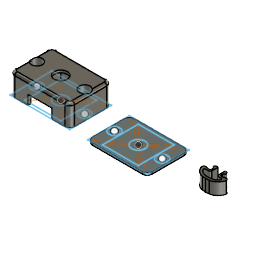
CNC Spindle speed control potentiometer box (Autodesk Fusion 360 design; units mm, degrees)
part number: 2025-11-11-00-48-20-010
Autodesk Fusion 360 part; units mm, degrees
other "Base Mesh Feature1"
sketch "Sketch1" plane through (0, 0, 0) normal (0, 0, 1) x (1, 0, 0)
other "Modify1"
sketch "Sketch2" plane through (0, 0, 0) normal (0, 0, 1) x (1, 0, 0)
  line L0 (5.2002, 7.2077) -> (5.2002, 2)
  line L1 (6.4101, 4.1476) -> (6.4101, 3)
  line L2 (11.227, 2.6891) -> (8.0821, 2.1867)
  spline S0 degree 5 poles (11.227, 2.6891) (11.2864, 2.6814) (11.4042, 2.6639) (11.5779, 2.6318) (11.8016, 2.5766) (12.0565, 2.4831) (12.2727, 2.3609) (12.4387, 2.206) (12.55, 2.0168) (12.6151, 1.7964) (12.65, 1.5503) (12.6682, 1.3375) (12.6829, 1.1712) (12.6941, 1.0575) (12.7, 1) knots 0 0 0 0 0 0 0.1 0.2 0.3 0.4 0.5 0.6 0.7 0.8 0.9 1 1 1 1 1 1
  spline S1 degree 5 poles (5.2002, 2) (5.2142, 1.9539) (5.2401, 1.8645) (5.2731, 1.7384) (5.3089, 1.585) (5.3615, 1.4113) (5.4474, 1.2482) (5.5895, 1.0908) (5.7997, 0.9399) (6.0785, 0.8015) (6.4184, 0.6836) (6.8058, 0.5942) (7.2236, 0.5392) (7.6535, 0.5196) (8.0779, 0.5294) (8.4811, 0.5571) (8.8496, 0.5877) (9.1727, 0.6054) (9.4429, 0.5948) (9.6569, 0.5437) (9.8164, 0.4447) (9.9265, 0.2963) (9.9931, 0.1031) (10.0203, -0.124) (10.0079, -0.3669) (9.9518, -0.6024) (9.867, -0.767) (9.7786, -0.8691) (9.7083, -0.9268) (9.6703, -0.953) knots 0 0 0 0 0 0 0.04 0.08 0.12 0.16 0.2 0.24 0.28 0.32 0.36 0.4 0.44 0.48 0.52 0.56 0.6 0.64 0.68 0.72 0.76 0.8 0.84 0.88 0.92 0.96 1 1 1 1 1 1
  spline S2 degree 5 poles (9.6703, -0.953) (9.6547, -0.9798) (9.622, -1.0343) (9.569, -1.1192) (9.4892, -1.2386) (9.3695, -1.4003) (9.2247, -1.5763) (9.0513, -1.7668) (8.8501, -1.9697) (8.625, -2.1809) (8.3817, -2.3946) (8.1265, -2.6048) (7.8654, -2.8053) (7.6023, -2.9907) (7.3391, -3.1569) (7.0767, -3.3009) (6.8155, -3.4216) (6.5564, -3.5198) (6.3019, -3.5984) (6.0562, -3.6628) (5.8229, -3.719) (5.6038, -3.7725) (5.3965, -3.8268) (5.192, -3.8817) (4.9756, -3.9335) (4.7324, -3.9774) (4.4506, -4.0091) (4.1264, -4.0264) (3.7682, -4.032) (3.394, -4.0317) (3.0255, -4.0329) (2.7526, -4.041) (2.5678, -4.0537) (2.4543, -4.0654) (2.4, -4.0721) knots 0 0 0 0 0 0 0.033333 0.066667 0.1 0.133333 0.166667 0.2 0.233333 0.266667 0.3 0.333333 0.366667 0.4 0.433333 0.466667 0.5 0.533333 0.566667 0.6 0.633333 0.666667 0.7 0.733333 0.766667 0.8 0.833333 0.866667 0.9 0.933333 0.966667 1 1 1 1 1 1
  spline S3 degree 5 poles (5.2002, 7.2077) (5.2051, 7.2204) (5.2155, 7.2451) (5.2328, 7.2805) (5.2591, 7.3248) (5.297, 7.3759) (5.3317, 7.4128) (5.3607, 7.4379) (5.3816, 7.4532) (5.3924, 7.4605) knots 0 0 0 0 0 0 0.2 0.4 0.6 0.8 1 1 1 1 1 1
  line L3 (5.3634, 7.4409) -> (5.4213, 7.4801)
  spline S4 degree 5 poles (5.3924, 7.4605) (5.4285, 7.472) (5.5013, 7.493) (5.6116, 7.5185) (5.761, 7.5402) (5.9516, 7.5467) (6.1454, 7.5323) (6.3417, 7.497) (6.539, 7.4417) (6.7351, 7.3677) (6.927, 7.2776) (7.1114, 7.1742) (7.2845, 7.0603) (7.4428, 6.9378) (7.5829, 6.8079) (7.7021, 6.67) (7.7983, 6.5221) (7.87, 6.3627) (7.9162, 6.1914) (7.9367, 6.0106) (7.932, 5.8267) (7.9028, 5.6507) (7.8507, 5.4947) (7.7772, 5.3684) (7.6837, 5.2758) (7.5716, 5.2119) (7.4419, 5.1603) (7.2966, 5.1006) (7.1386, 5.0134) (6.9737, 4.8869) (6.8104, 4.7224) (6.6611, 4.5394) (6.5384, 4.3652) (6.4522, 4.2273) (6.4066, 4.1444) (6.3971, 4.1188) (6.4045, 4.1238) (6.4089, 4.1259) (6.41, 4.1239) (6.4101, 4.1221) knots 0 0 0 0 0 0 0.028571 0.057143 0.085714 0.114286 0.142857 0.171429 0.2 0.228571 0.257143 0.285714 0.314286 0.342857 0.371429 0.4 0.428571 0.457143 0.485714 0.514286 0.542857 0.571429 0.6 0.628571 0.657143 0.685714 0.714286 0.742857 0.771429 0.8 0.828571 0.857143 0.885714 0.914286 0.942857 0.971429 1 1 1 1 1 1
  line L4 (6.396, 4.6404) -> (6.4241, 3.6037)
  spline S5 degree 5 poles (6.4101, 3) (6.4295, 2.9151) (6.482, 2.7582) (6.6016, 2.5616) (6.8341, 2.3729) (7.1978, 2.2388) (7.5745, 2.1806) (7.9066, 2.1719) (8.1517, 2.1888) (8.2998, 2.2137) (8.3827, 2.237) (8.4352, 2.2507) (8.4872, 2.2577) (8.5305, 2.2609) (8.5542, 2.2622) knots 0 0 0 0 0 0 0.1 0.2 0.3 0.4 0.5 0.6 0.7 0.8 0.9 1 1 1 1 1 1
  line L5 (8.3639, 2.2523) -> (8.7446, 2.2721)
  spline S6 degree 5 poles (12.7, 1) (12.6553, 0.8629) (12.5632, 0.5911) (12.4169, 0.1912) (12.2038, -0.3275) (11.8989, -0.9549) (11.5457, -1.5648) (11.1367, -2.159) (10.6703, -2.7361) (10.1549, -3.2896) (9.6039, -3.8101) (9.0321, -4.2869) (8.451, -4.7097) (7.8653, -5.0706) (7.268, -5.3665) (6.6441, -5.5977) (6.1102, -5.7322) (5.6836, -5.8056) (5.3868, -5.8426) (5.2352, -5.858) knots 0 0 0 0 0 0 0.066667 0.133333 0.2 0.266667 0.333333 0.4 0.466667 0.533333 0.6 0.666667 0.733333 0.8 0.866667 0.933333 1 1 1 1 1 1
  line L6 (6.4983, -5.7292) -> (3.9722, -5.9869)
  line L7 (2.4, 20) -> (2.4, -85)
  spline S7 degree 5 poles (-6.427, 2.6891) (-6.4864, 2.6814) (-6.6042, 2.6639) (-6.7779, 2.6318) (-7.0016, 2.5766) (-7.2565, 2.4831) (-7.4727, 2.3609) (-7.6387, 2.206) (-7.75, 2.0168) (-7.8151, 1.7964) (-7.85, 1.5503) (-7.8682, 1.3375) (-7.8829, 1.1712) (-7.8941, 1.0575) (-7.9, 1) knots 0 0 0 0 0 0 0.1 0.2 0.3 0.4 0.5 0.6 0.7 0.8 0.9 1 1 1 1 1 1
  line L8 (11.0149, 2.7167) -> (11.4391, 2.6615)
  line L9 (12.6774, 1.2187) -> (12.7226, 0.7813)
  line L10 (-6.2149, 2.7167) -> (-6.6391, 2.6615)
  line L11 (-7.8774, 1.2187) -> (-7.9226, 0.7813)
  spline S8 degree 5 poles (-0.5924, 7.4605) (-0.6285, 7.472) (-0.7013, 7.493) (-0.8116, 7.5185) (-0.961, 7.5402) (-1.1516, 7.5467) (-1.3454, 7.5323) (-1.5417, 7.497) (-1.739, 7.4417) (-1.9351, 7.3677) (-2.127, 7.2776) (-2.3114, 7.1742) (-2.4845, 7.0603) (-2.6428, 6.9378) (-2.7829, 6.8079) (-2.9021, 6.67) (-2.9983, 6.5221) (-3.07, 6.3627) (-3.1162, 6.1914) (-3.1367, 6.0106) (-3.132, 5.8267) (-3.1028, 5.6507) (-3.0507, 5.4947) (-2.9772, 5.3684) (-2.8837, 5.2758) (-2.7716, 5.2119) (-2.6419, 5.1603) (-2.4966, 5.1006) (-2.3386, 5.0134) (-2.1737, 4.8869) (-2.0104, 4.7224) (-1.8611, 4.5394) (-1.7384, 4.3652) (-1.6522, 4.2273) (-1.6066, 4.1444) (-1.5971, 4.1188) (-1.6045, 4.1238) (-1.6089, 4.1259) (-1.61, 4.1239) (-1.6101, 4.1221) knots 0 0 0 0 0 0 0.028571 0.057143 0.085714 0.114286 0.142857 0.171429 0.2 0.228571 0.257143 0.285714 0.314286 0.342857 0.371429 0.4 0.428571 0.457143 0.485714 0.514286 0.542857 0.571429 0.6 0.628571 0.657143 0.685714 0.714286 0.742857 0.771429 0.8 0.828571 0.857143 0.885714 0.914286 0.942857 0.971429 1 1 1 1 1 1
  line L12 (4.9117, 7.3077) -> (5.873, 7.6134)
  line L13 (-0.1117, 7.3077) -> (-1.073, 7.6134)
  line L14 (-1.596, 4.6404) -> (-1.6241, 3.6037)
  line L15 (-1.6101, 4.1476) -> (-1.6101, 3)
  spline S9 degree 5 poles (-7.9, 1) (-7.8553, 0.8629) (-7.7632, 0.5911) (-7.6169, 0.1912) (-7.4038, -0.3275) (-7.0989, -0.9549) (-6.7457, -1.5648) (-6.3367, -2.159) (-5.8703, -2.7361) (-5.3549, -3.2896) (-4.8039, -3.8101) (-4.2321, -4.2869) (-3.651, -4.7097) (-3.0653, -5.0706) (-2.468, -5.3665) (-1.8441, -5.5977) (-1.3102, -5.7322) (-0.8836, -5.8056) (-0.5868, -5.8426) (-0.4352, -5.858) knots 0 0 0 0 0 0 0.066667 0.133333 0.2 0.266667 0.333333 0.4 0.466667 0.533333 0.6 0.666667 0.733333 0.8 0.866667 0.933333 1 1 1 1 1 1
  line L16 (13.0643, 2.1177) -> (12.3357, -0.1177)
  line L17 (-8.2643, 2.1177) -> (-7.5357, -0.1177)
  line L18 (-1.6983, -5.7292) -> (0.8278, -5.9869)
  line L19 (-0.4002, 7.2077) -> (-0.4002, 2)
  spline S10 degree 5 poles (-1.6101, 3) (-1.6295, 2.9151) (-1.682, 2.7582) (-1.8016, 2.5616) (-2.0341, 2.3729) (-2.3978, 2.2388) (-2.7745, 2.1806) (-3.1066, 2.1719) (-3.3517, 2.1888) (-3.4998, 2.2137) (-3.5827, 2.237) (-3.6352, 2.2507) (-3.6872, 2.2577) (-3.7305, 2.2609) (-3.7542, 2.2622) knots 0 0 0 0 0 0 0.1 0.2 0.3 0.4 0.5 0.6 0.7 0.8 0.9 1 1 1 1 1 1
  line L20 (6.3637, 3.2024) -> (6.4564, 2.7976)
  line L21 (-1.5637, 3.2024) -> (-1.6564, 2.7976)
  line L22 (-3.5639, 2.2523) -> (-3.9446, 2.2721)
  spline S11 degree 5 poles (-0.4002, 7.2077) (-0.4051, 7.2204) (-0.4155, 7.2451) (-0.4328, 7.2805) (-0.4591, 7.3248) (-0.497, 7.3759) (-0.5317, 7.4128) (-0.5607, 7.4379) (-0.5816, 7.4532) (-0.5924, 7.4605) knots 0 0 0 0 0 0 0.2 0.4 0.6 0.8 1 1 1 1 1 1
  line L23 (5.1871, 7.1737) -> (5.2134, 7.2418)
  line L24 (-0.3871, 7.1737) -> (-0.4134, 7.2418)
  line L25 (-0.5634, 7.4409) -> (-0.6213, 7.4801)
  spline S12 degree 5 poles (-0.4002, 2) (-0.4142, 1.9539) (-0.4401, 1.8645) (-0.4731, 1.7384) (-0.5089, 1.585) (-0.5615, 1.4113) (-0.6474, 1.2482) (-0.7895, 1.0908) (-0.9997, 0.9399) (-1.2785, 0.8015) (-1.6184, 0.6836) (-2.0058, 0.5942) (-2.4236, 0.5392) (-2.8535, 0.5196) (-3.2779, 0.5294) (-3.6811, 0.5571) (-4.0496, 0.5877) (-4.3727, 0.6054) (-4.6429, 0.5948) (-4.8569, 0.5437) (-5.0164, 0.4447) (-5.1265, 0.2963) (-5.1931, 0.1031) (-5.2203, -0.124) (-5.2079, -0.3669) (-5.1518, -0.6024) (-5.067, -0.767) (-4.9786, -0.8691) (-4.9083, -0.9268) (-4.8703, -0.953) knots 0 0 0 0 0 0 0.04 0.08 0.12 0.16 0.2 0.24 0.28 0.32 0.36 0.4 0.44 0.48 0.52 0.56 0.6 0.64 0.68 0.72 0.76 0.8 0.84 0.88 0.92 0.96 1 1 1 1 1 1
  line L26 (4.9603, 2.7917) -> (5.4402, 1.2083)
  line L27 (10.2043, -0.5845) -> (9.1364, -1.3215)
  line L28 (-0.1603, 2.7917) -> (-0.6402, 1.2083)
  line L29 (-5.4043, -0.5845) -> (-4.3364, -1.3215)
  spline S13 degree 5 poles (-4.8703, -0.953) (-4.8547, -0.9798) (-4.822, -1.0343) (-4.769, -1.1192) (-4.6892, -1.2386) (-4.5695, -1.4003) (-4.4247, -1.5763) (-4.2513, -1.7668) (-4.0501, -1.9697) (-3.825, -2.1809) (-3.5817, -2.3946) (-3.3265, -2.6048) (-3.0654, -2.8053) (-2.8023, -2.9907) (-2.5391, -3.1569) (-2.2767, -3.3009) (-2.0155, -3.4216) (-1.7564, -3.5198) (-1.5019, -3.5984) (-1.2562, -3.6628) (-1.0229, -3.719) (-0.8038, -3.7725) (-0.5965, -3.8268) (-0.392, -3.8817) (-0.1756, -3.9335) (0.0676, -3.9774) (0.3494, -4.0091) (0.6736, -4.0264) (1.0318, -4.032) (1.406, -4.0317) (1.7745, -4.0329) (2.0474, -4.041) (2.2322, -4.0537) (2.3457, -4.0654) (2.4, -4.0721) knots 0 0 0 0 0 0 0.033333 0.066667 0.1 0.133333 0.166667 0.2 0.233333 0.266667 0.3 0.333333 0.366667 0.4 0.433333 0.466667 0.5 0.533333 0.566667 0.6 0.633333 0.666667 0.7 0.733333 0.766667 0.8 0.833333 0.866667 0.9 0.933333 0.966667 1 1 1 1 1 1
  line L30 (10.0011, -0.3866) -> (9.3396, -1.5194)
  line L31 (3.0554, -3.9915) -> (1.7446, -4.1527)
  line L32 (-5.2011, -0.3866) -> (-4.5396, -1.5194)
  line L33 (1.7446, -3.9915) -> (3.0554, -4.1527)
  line L34 (-6.427, 2.6891) -> (-3.2821, 2.1867)
  line L35 (5.2352, -5.858) -> (2.4, -6.1473)
  line L36 (-0.4352, -5.858) -> (2.4, -6.1473)
  point P0 (6.4628, 7.4605)
  point P1 (7.5078, 6.8743)
  point P2 (7.9283, 6.046)
  point P3 (7.7, 5.3)
  point P4 (7, 4.9)
  point P5 (12.4313, 2.1898)
  point P6 (11.1293, -2.1455)
  point P7 (8.378, -4.7419)
  point P8 (5.5, 1.2)
  point P9 (7.2619, 0.545)
  point P10 (9.4941, 0.5743)
  point P11 (10, 0)
  point P12 (9.2, -1.6)
  point P13 (8, -2.7)
  point P14 (6.6, -3.5)
  point P15 (5.5, -3.8)
  point P16 (4.3928, -4.0092)
  point P17 (-7.6313, 2.1898)
  point P18 (-4.6941, 0.5743)
  point P19 (-5.2, 0)
  point P20 (-2.9, 5.3)
  point P21 (-2.4619, 0.545)
  point P22 (-6.3293, -2.1455)
  point P23 (-0.7, 1.2)
  point P24 (-1.6628, 7.4605)
  point P25 (-3.578, -4.7419)
  point P26 (-4.4, -1.6)
  point P27 (-2.2, 4.9)
  point P28 (-3.1283, 6.046)
  point P29 (-1.8, -3.5)
  point P30 (-2.7078, 6.8743)
  point P31 (-0.7, -3.8)
  point P32 (-3.2, -2.7)
  point P33 (0.4072, -4.0092)
  constraint coincident S3.end S4.start
  constraint midpoint S3.end L3
  constraint coincident L1 S4.end
  constraint midpoint S4.end L4
  constraint coincident L2 S5.end
  constraint midpoint S5.end L5
  constraint midpoint S6.end L6
  constraint midpoint L2.start L8
  constraint midpoint S0.end L9
  constraint midpoint S3.end L12
  constraint midpoint S0.end L16
  constraint midpoint L1.end L20
  constraint midpoint L0.start L23
  constraint midpoint L0.end L26
  constraint midpoint S1.end L27
  constraint midpoint S1.end L30
  constraint midpoint S2.end L31
  constraint symmetric L0.start L7 L19.start
  constraint symmetric L0.end L7 L19.end
  constraint symmetric L1.start L7 L15.start
  constraint symmetric L1.end L7 L15.end
  constraint symmetric L2.start L7 S7.start
  constraint symmetric L2.end L7 L34.end
  constraint symmetric S3.end L7 S8.start
  constraint symmetric P0 L7 P24
  constraint symmetric P1 L7 P30
  constraint symmetric P2 L7 P28
  constraint symmetric P3 L7 P20
  constraint symmetric P4 L7 P27
  constraint symmetric P5 L7 P17
  constraint symmetric S0.end L7 S7.end
  constraint symmetric P6 L7 P22
  constraint symmetric P7 L7 P25
  constraint symmetric P8 L7 P23
  constraint symmetric P9 L7 P21
  constraint symmetric P10 L7 P18
  constraint symmetric P11 L7 P19
  constraint symmetric S1.end L7 S12.end
  constraint symmetric P12 L7 P26
  constraint symmetric P13 L7 P32
  constraint symmetric P14 L7 P29
  constraint symmetric P15 L7 P31
  constraint symmetric P16 L7 P33
  constraint symmetric L3.start L7 L25.start
  constraint symmetric L3.end L7 L25.end
  constraint symmetric S4.end L7 S8.end
  constraint symmetric L4.start L7 L14.start
  constraint symmetric L4.end L7 L14.end
  constraint symmetric S5.end L7 S10.end
  constraint symmetric L5.start L7 L22.start
  constraint symmetric L5.end L7 L22.end
  constraint symmetric S6.end L7 S9.end
  constraint symmetric L6.start L7 L18.start
  constraint symmetric L6.end L7 L18.end
  constraint symmetric L7 L8.start L10.start
  constraint symmetric L7 L8.end L10.end
  constraint symmetric L7 L9.start L11.start
  constraint symmetric L7 L9.end L11.end
  constraint symmetric L7 L12.start L13.start
  constraint symmetric L7 L12.end L13.end
  constraint symmetric L7 L16.start L17.start
  constraint symmetric L7 L16.end L17.end
  constraint symmetric L7 L20.start L21.start
  constraint symmetric L7 L20.end L21.end
  constraint symmetric L7 L23.start L24.start
  constraint symmetric L7 L23.end L24.end
  constraint symmetric L7 L26.start L28.start
  constraint symmetric L7 L26.end L28.end
  constraint symmetric L7 L27.start L29.start
  constraint symmetric L7 L27.end L29.end
  constraint symmetric L7 L30.start L32.start
  constraint symmetric L7 L30.end L32.end
  constraint symmetric L7 L31.start L33.start
  constraint symmetric L7 L31.end L33.end
  constraint coincident L7 L35.end
extrude "Extrude5" add sketch "Sketch2" along normal blind 10 contours L0 L1 L2 S0 S1 S2 S3 L3 S4 S5 S6 L6 L7 L9 L23 L26 L35 | S1 L26 | L7 S7 L11 S8 L15 S9 L18 L19 S10 S11 L24 L25 S12 L28 S13 L34 L36 | S12 L28 makes body 1
sketch "Sketch5" plane through (0, 0, 0) normal (0, 0, 1) x (1, 0, 0)
  circle A0 centre (-60, 0) radius 5.5
  line L0 (-35, 17.5) -> (-85, 17.5)
  line L1 (-85, 17.5) -> (-85, -17.5)
  line L2 (-85, -17.5) -> (-35, -17.5)
  line L3 (-35, -17.5) -> (-35, 17.5)
  line L4 (-35, 17.5) -> (-85, -17.5) construction
  line L5 (-85, 17.5) -> (-35, -17.5) construction
  line L6 (-45, 15) -> (-75, 15)
  line L7 (-75, 15) -> (-75, -15)
  line L8 (-75, -15) -> (-45, -15)
  line L9 (-45, -15) -> (-45, 15)
  line L10 (-45, 15) -> (-75, -15) construction
  line L11 (-75, 15) -> (-45, -15) construction
  circle A1 centre (-40, 0) radius 4.5
  circle A2 centre (-80, 0) radius 4.5
  circle A3 centre (-40, 0) radius 2.75
  circle A4 centre (-80, 0) radius 2.75
  circle A5 centre (-105, 0) radius 2.75
  line L12 (-140, -15) -> (-110, -15)
  circle A6 centre (-125, 0) radius 5.5
  line L13 (-140, 15) -> (-140, -15)
  line L14 (-100, 17.5) -> (-150, 17.5)
  line L15 (-110, 15) -> (-140, -15) construction
  circle A7 centre (-145, 0) radius 4.5
  line L16 (-150, 17.5) -> (-150, -17.5)
  line L17 (-100, 17.5) -> (-150, -17.5) construction
  line L18 (-140, 15) -> (-110, -15) construction
  line L19 (-100, -17.5) -> (-100, 17.5)
  line L20 (-110, 15) -> (-140, 15)
  circle A8 centre (-145, 0) radius 2.75
  line L21 (-110, -15) -> (-110, 15)
  line L22 (-150, -17.5) -> (-100, -17.5)
  circle A9 centre (-105, 0) radius 4.5
  line L23 (-150, 17.5) -> (-100, -17.5) construction
  point P0 (-60, 0)
  point P1 (-60, 0)
  point P2 (-125, 0)
  point P3 (-125, 0)
  dimension "d22" = 11
  dimension "d23" = 50
  dimension "d24" = 35
  dimension "d25" = 30
  dimension "d26" = 30
  dimension "d27" = 9
  dimension "d28" = 9
  dimension "d29" = 5.5
  dimension "d30" = 5.5
  dimension "d33" = 11
  dimension "d34" = 50
  dimension "d35" = 35
  dimension "d36" = 30
  dimension "d37" = 30
  dimension "d38" = 9
  dimension "d39" = 9
  dimension "d40" = 5.5
  dimension "d41" = 5.5
  constraint horizontal L0
  constraint perpendicular L0 L1
  constraint parallel L0 L2
  constraint parallel L1 L3
  constraint coincident L4 P1
  constraint coincident L5 P1
  constraint coincident P0 A0.centre
  constraint horizontal L6
  constraint perpendicular L6 L7
  constraint parallel L6 L8
  constraint parallel L7 L9
  constraint coincident L10 P1
  constraint coincident L11 P1
  constraint concentric A1 A3
  constraint concentric A2 A4
  constraint horizontal L14
  constraint perpendicular L14 L16
  constraint parallel L14 L22
  constraint parallel L16 L19
  constraint coincident P3 L17
  constraint coincident P3 L23
  constraint coincident P3 P2
  constraint horizontal L20
  constraint perpendicular L13 L20
  constraint parallel L12 L20
  constraint parallel L13 L21
  constraint coincident P3 L15
  constraint coincident P3 L18
  constraint concentric A5 A9
  constraint concentric A7 A8
  measures "d22" diameter of A0
  measures "d23" distance of L1.end L2.end
  measures "d24" distance of L0.end L1.end
  measures "d25" distance of L7.end L8.end
  measures "d26" distance of L6.end L7.end
  measures "d27" diameter of A1
  measures "d28" diameter of A2
  measures "d29" diameter of A3
  measures "d30" diameter of A4
  measures "d33" diameter of A6
  measures "d34" distance of L16.end L19.start
  measures "d35" distance of L16.end L14.end
  measures "d36" distance of L12.start L12.end
  measures "d37" distance of L12.start L13.start
  measures "d38" diameter of A9
  measures "d39" diameter of A7
  measures "d40" diameter of A5
  measures "d41" diameter of A8
extrude "Extrude6" add sketch "Sketch5" against normal blind 2 separate body contours A0 | L0 L1 L2 L3 | L6 L7 L8 L9 | A1 | A2 makes body 2
extrude "Extrude7" add sketch "Sketch5" along normal blind 18 separate body contours L12 L13 L20 L21 | L14 L16 L19 L22 | A7 | A9 makes body 3
extrude "Extrude8" cut sketch "Sketch5" along normal blind 12 contours L12 L13 L20 L21 bodies 3
sketch "Sketch6" plane through (0, 0, 18) normal (0, 0, 1) x (-1, 0, 0)
  circle A0 centre (125, 0) radius 5.5
  circle A1 centre (105, 0) radius 2.75
  circle A2 centre (145, 0) radius 2.75
  line L0 (150, 17.5) -> (100, 17.5)
  line L1 (100, 17.5) -> (100, -17.5)
  line L2 (100, -17.5) -> (150, -17.5)
  line L3 (150, -17.5) -> (150, 17.5)
  circle A3 centre (105, 0) radius 4.5
  circle A4 centre (145, 0) radius 4.5
  dimension "d46" = 9
  dimension "d47" = 9
  constraint concentric A1 A3
  constraint concentric A2 A4
  measures "d46" diameter of A3
  measures "d47" diameter of A4
extrude "Extrude9" cut sketch "Sketch6" against normal blind 8 contours A3 | A4 bodies 3
sketch "Sketch7" plane through (0, -17.5, 0) normal (0, -1, 0) x (1, 0, 0)
  line L0 (-150, 0) -> (-100, 0)
  line L1 (-100, 0) -> (-100, 18)
  line L2 (-100, 18) -> (-150, 18)
  line L3 (-150, 18) -> (-150, 0)
  line L4 (-115, 8) -> (-135, 8)
  line L5 (-135, 8) -> (-135, -12)
  line L6 (-135, -12) -> (-115, -12)
  line L7 (-115, -12) -> (-115, 8)
  point P0 (-125, 7)
  dimension "d50" = 20
  constraint perpendicular L4 L5
  measures "d50" distance of L4.end L5.end
extrude "Extrude10" cut sketch "Sketch7" against normal blind 4 contours L0 L4 L5 L7 bodies 3
fillet "Fillet6" radius 4 1 edges at (-100, -17.5, 9) on bodies 3
fillet "Fillet7" radius 4 3 edges at (-100, 17.5, 9) (-150, -17.5, 9) (-150, 17.5, 9) on bodies 3
fillet "Fillet8" radius 2 8 edges at (-148.8284, -16.3284, 18) (-125, -17.5, 18) (-101.1716, -16.3284, 18) (-100, 0, 18) (-101.1716, 16.3284, 18) (-125, 17.5, 18) (-148.8284, 16.3284, 18) (-150, 0, 18) on bodies 3
fillet "Fillet9" radius 4 4 edges at (-85, 17.5, -1) (-35, 17.5, -1) (-35, -17.5, -1) (-85, -17.5, -1) on bodies 2
extrude "Extrude11" cut 1 faces at (-125.137, 11.8282, 12) along direction (0, 0, 1) blind 4 on bodies 3 bodies 3
